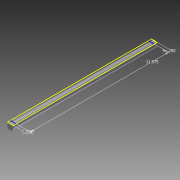
# Autodesk Inventor part: 8 ball roller shaft
Saved by Autodesk Inventor 2012 (Build 160160000, 160)
## iProperties
Created: 2013-11-12
Part Number: 8 ball roller shaft
Material: Default
Document SubType Name: Modeling
Designer: Bryce
Density: 1 g/cm^3
Author: Bryce
Autodesk Inventor part; units mm, degrees
ref_plane "YZ Plane" through (0, 0, 0) normal (1, 0, 0) x (0, 1, 0)
ref_plane "XY Plane" through (0, 0, 0) normal (0, 0, 1) x (1, 0, 0)
sketch "Sketch1" plane through (0, 0, 0) normal (0, 0, 1) x (1, 0, 0)
  circle A0 centre (0, 0) radius 6.35
  dimension "d0" = 12.7
  constraints: 1 centre point, 1 coincident
  measures "d0" diameter of A0
extrude "Extrusion1" add sketch "Sketch1" along normal blind 314.325
ref_plane "Work Plane1" through (0, 6.35, 0) normal (0, 1, 0) x (-1, 0, 0)
sketch "Sketch2" plane through (0, 6.35, 0) normal (0, 1, 0) x (-1, 0, 0)
  line L0 (-6.35, 314.325) -> (6.35, 314.325) projected
  line L1 (-6.35, 0) -> (6.35, 0) projected
  line L2 (-6.35, 0) -> (-6.35, 314.325) projected
  line L3 (6.35, 0) -> (6.35, 314.325) projected
  line L4 (-6.35, 6.35) -> (6.35, 6.35)
  line L5 (-6.35, 307.975) -> (6.35, 307.975)
  point P0 (0, 0)
  dimension "d3" = 301.625
  dimension "d4" = 6.35
  dimension "d5" = 6.35
  constraints: 4 end point, 4 point on line, 2 perpendicular
  measures "d3" distance between parallel lines of L4 L5
  measures "d4" distance between parallel lines of L1 L4
  measures "d5" distance between parallel lines of L0 L5
ref_plane "Work Plane2" through (6.35, 6.35, 307.975) normal (0, 0, 1) x (1, 0, 0)
ref_plane "Work Plane3" through (6.35, 6.35, 6.35) normal (0, 0, -1) x (-1, 0, 0)
sketch "Sketch3" plane through (6.35, 6.35, 307.975) normal (0, 0, 1) x (1, 0, 0)
  circle A0 centre (-6.35, -6.35) radius 6.35 projected
  circle A1 centre (-6.35, -6.35) radius 5.08
  dimension "d6" = 10.16
  constraints: 1 centre point, 1 coincident
  measures "d6" diameter of A1
extrude "Extrusion2" cut sketch "Sketch3" against normal blind 1.016
sketch "Sketch4" plane through (6.35, 6.35, 6.35) normal (0, 0, -1) x (-1, 0, 0)
  circle A0 centre (6.35, -6.35) radius 5.08 projected
  circle A1 centre (6.35, -6.35) radius 6.35 projected
extrude "Extrusion3" cut sketch "Sketch4" against normal blind 1.016
equation "\"d4\" = d5"
body "Solid1"
